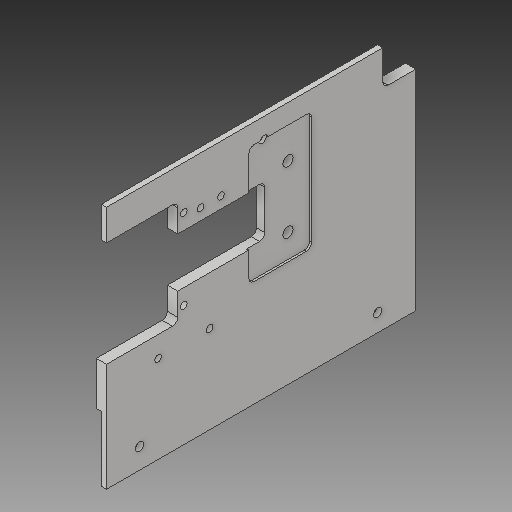
# Autodesk Inventor part: DriveSideBallScrewSupport
Saved by Autodesk Inventor 2018 (Build 220112000, 112)
## iProperties
Created: 2017-10-24
Part Number: DriveSideBallScrewSupport
Material: Generic
Document SubType Name: Modeling
Designer: m228540
Density: 1 g/cm^3
Appearance: Default
Author: m228540
Autodesk Inventor part; units mm, degrees
ref_plane "YZ Plane" through (0, 0, 0) normal (1, 0, 0) x (0, 1, 0)
ref_plane "XZ Plane" through (0, 0, 0) normal (0, 1, 0) x (-1, 0, 0)
ref_plane "XY Plane" through (0, 0, 0) normal (0, 0, 1) x (1, 0, 0)
sketch "Sketch1" plane through (0, 0, 0) normal (1, 0, 0) x (0, 1, 0)
  line L0 (118.5, 150) -> (-118.5, 150)
  line L1 (-118.5, 150) -> (-118.5, -150)
  line L2 (-118.5, -150) -> (118.5, -150)
  line L3 (118.5, -150) -> (118.5, 150)
  line L4 (118.5, 150) -> (-118.5, -150) construction
  line L5 (-118.5, 150) -> (118.5, -150) construction
  point P0 (0, 0)
  dimension "d0" = 300
  dimension "d1" = 237
  constraints: 12 end point, 2 midpoint, 2 parallel, 1 horizontal, 1 perpendicular
  measures "d0" distance of L0.end L1.end
  measures "d1" distance of L1.end L2.end
extrude "Extrusion1" add sketch "Sketch1" along normal mid plane 10
sketch "Sketch2" plane through (5, 0, 0) normal (1, 0, 0) x (0, 0, -1)
  line L0 (150, -118.5) -> (150, 118.5) projected
  line L1 (150, 118.5) -> (118, 118.5)
  line L2 (118, 118.5) -> (118, 89.5)
  line L3 (123, 84.5) -> (150, 84.5)
  line L4 (150, 84.5) -> (150, 118.5)
  arc A0 (118, 89.5) -> (123, 84.5) centre (123, 89.5) ccw
  point P0 (0, 0)
  point P1 (118, 84.5)
  dimension "d4" = 32
  dimension "d5" = 34
  dimension "d6" = 5
  constraints: 8 end point, 2 parallel, 2 point on circle, 2 point on line, 2 tangent, 1 centre point, 1 horizontal, 1 perpendicular
  measures "d4" distance of point (118, 84.5) L3.end
  measures "d5" distance of L1.end point (118, 84.5)
  measures "d6" radius of A0
extrude "Extrusion2" cut sketch "Sketch2" against normal through all
sketch "Sketch3" plane through (5, 0, 0) normal (1, 0, 0) x (0, 0, -1)
  line L0 (-7, -15.5) -> (44, -15.5)
  line L1 (49, -10.5) -> (49, 94.5)
  line L2 (44, 99.5) -> (-7, 99.5)
  line L3 (-12, 94.5) -> (-12, -10.5)
  line L4 (-12, -15.5) -> (49, 99.5) construction
  line L5 (49, -15.5) -> (-12, 99.5) construction
  line L6 (-150, 118.5) -> (-150, -118.5) projected
  line L7 (118, 118.5) -> (-150, 118.5) projected
  arc A0 (-7, 99.5) -> (-12, 94.5) centre (-7, 94.5) ccw
  arc A1 (49, 94.5) -> (44, 99.5) centre (44, 94.5) ccw
  arc A2 (44, -15.5) -> (49, -10.5) centre (44, -10.5) ccw
  arc A3 (-12, -10.5) -> (-7, -15.5) centre (-7, -10.5) ccw
  point P0 (0, 0)
  point P1 (18.5, 42)
  dimension "d9" = 138
  dimension "d10" = 115
  dimension "d11" = 61
  dimension "d12" = 19
  dimension "d13" = 5
  constraints: 12 end point, 8 point on circle, 8 point on line, 8 tangent, 4 centre point, 3 equal radius, 2 midpoint, 2 parallel, 1 horizontal, 1 perpendicular
  measures "d9" distance between parallel lines of L6 L3
  measures "d10" distance of L5.end L4.start
  measures "d11" distance of L4.end L5.end
  measures "d12" distance between parallel lines of L7 L2
  measures "d13" radius of A0
extrude "Extrusion3" cut sketch "Sketch3" against normal blind 2
sketch "Sketch4" plane through (5, 0, 0) normal (1, 0, 0) x (0, 0, -1)
  circle A0 centre (-118, -98.5) radius 4
  circle A1 centre (113, -101.5) radius 4
  circle A2 centre (3, 98.5) radius 4
  line L0 (-150, -118.5) -> (-150, 118.5) projected
  line L1 (-150, -118.5) -> (150, -118.5) projected
  line L2 (150, -118.5) -> (150, 84.5) projected
  line L3 (118, 118.5) -> (-150, 118.5) projected
  point P0 (0, 0)
  dimension "d16" = 8
  dimension "d17" = 32
  dimension "d18" = 20
  dimension "d19" = 17
  dimension "d20" = 37
  dimension "d21" = 153
  dimension "d22" = 20
  constraints: 3 centre point, 2 equal radius
  measures "d16" diameter of A0
  measures "d17" distance from line of L0 A0.centre
  measures "d18" distance from line of L1 A0.centre
  measures "d19" distance from line of L1 A1.centre
  measures "d20" distance from line of L2 A1.centre
  measures "d21" distance from line of L0 A2.centre
  measures "d22" distance from line of L3 A2.centre
extrude "Extrusion4" cut sketch "Sketch4" against normal through all
sketch "Sketch5" plane through (-5, 0, 0) normal (-1, 0, 0) x (0, 0, 1)
  line L0 (150, -118.5) -> (-150, -118.5) projected
  line L1 (-150, -118.5) -> (-83, -118.5)
  line L2 (-83, -118.5) -> (-83, -55.5)
  line L3 (-83, -55.5) -> (-150, -55.5)
  line L4 (-150, -55.5) -> (-150, -118.5)
  line L5 (150, -118.5) -> (80, -118.5)
  line L6 (80, -118.5) -> (80, -55.5)
  line L7 (80, -55.5) -> (150, -55.5)
  line L8 (150, -55.5) -> (150, -118.5)
  line L9 (-118, 118.5) -> (150, 118.5) projected
  line L10 (-150, 84.5) -> (-123, 84.5) projected
  line L11 (150, 118.5) -> (-123, 118.5)
  line L12 (-123, 118.5) -> (-123, 84.5)
  line L13 (-123, 84.5) -> (150, 84.5)
  line L14 (150, 84.5) -> (150, 118.5)
  point P0 (0, 0)
  dimension "d25" = 70
  dimension "d26" = 63
  dimension "d27" = 63
  dimension "d28" = 67
  constraints: 24 end point, 6 parallel, 3 horizontal, 3 perpendicular
  measures "d25" distance of L6.end L7.end
  measures "d26" distance of L5.end L6.end
  measures "d27" distance of L1.end L2.end
  measures "d28" distance of L2.end L3.end
extrude "Extrusion5" cut sketch "Sketch5" against normal blind 5
sketch "Sketch6" plane through (3, 0, 0) normal (1, 0, 0) x (0, 0, -1)
  circle A0 centre (28, 67.5) radius 5
  circle A1 centre (28, 7.5) radius 5
  line L0 (150, -118.5) -> (150, 84.5) projected
  line L1 (118, 118.5) -> (-150, 118.5) projected
  point P0 (0, 0)
  dimension "d31" = 122
  dimension "d32" = 10
  dimension "d34" = 60
  dimension "d35" = 51
  constraints: 2 centre point, 1 equal radius, 1 vertical alignment
  measures "d31" distance from line of L0 A0.centre
  measures "d32" diameter of A0
  measures "d34" distance of A1.centre A0.centre
  measures "d35" distance from line of L1 A0.centre
extrude "Extrusion6" cut sketch "Sketch6" against normal through all
fillet "Fillet1" radius 5 2 edges at (-2.5, -55.5, 80) (-2.5, -55.5, -83)
sketch "Sketch7" plane through (5, 0, 0) normal (1, 0, 0) x (0, 0, -1)
  line L0 (-150, 118.5) -> (-150, -118.5) projected
  line L1 (-150, 88.5) -> (-81, 88.5)
  line L2 (-81, -13.5) -> (-150, -13.5)
  line L3 (-150, -13.5) -> (-150, 88.5)
  line L4 (118, 118.5) -> (-150, 118.5) projected
  line L5 (-81, 102.5) -> (-81, 62.1221) projected
  line L6 (-69, 62.1221) -> (-69, 102.5) projected
  line L7 (15.5, -2.5) -> (15.5, 77.5) projected
  line L8 (-81, 61.5) -> (5.5, 61.5)
  line L9 (5.5, 61.5) -> (5.5, 13.5)
  line L10 (5.5, 13.5) -> (-81, 13.5)
  line L11 (-81, 88.5) -> (-81, 61.5)
  line L12 (-81, 13.5) -> (-81, -13.5)
  point P0 (0, 0)
  dimension "d39" = 30
  dimension "d40" = 102
  dimension "d41" = 57
  dimension "d42" = 10
  dimension "d43" = 48
  constraints: 16 end point, 4 parallel, 3 perpendicular, 2 collinear, 2 horizontal, 2 point on line
  measures "d39" distance between parallel lines of L4 L1
  measures "d40" distance of L1.end L2.start
  measures "d41" distance between parallel lines of L8 L4
  measures "d42" distance between parallel lines of L9 L7
  measures "d43" distance of L8.end L9.end
extrude "Extrusion7" cut sketch "Sketch7" against normal through all
fillet "Fillet2" radius 5 4 edges at (2.5, 88.5, 81) (0, -13.5, 81) (-1, 13.5, -5.5) (-1, 61.5, -5.5)
sketch "Sketch8" plane through (5, 0, 0) normal (1, 0, 0) x (0, 0, -1)
  circle A0 centre (-100, -33.5) radius 3 construction
  circle A1 centre (-50, -33.5) radius 3 construction
  circle A2 centre (-59, 72.5) radius 3 construction
  circle A3 centre (-39, 72.5) radius 3 construction
  circle A4 centre (-75, 76.5) radius 3 construction
  circle A5 centre (-75, -1.5) radius 3 construction
  circle A6 centre (-75, 76.5) radius 3.25
  circle A7 centre (-59, 72.5) radius 3.25
  circle A8 centre (-39, 72.5) radius 3.25
  circle A9 centre (-75, -1.5) radius 3.25
  circle A10 centre (-50, -33.5) radius 3.25
  circle A11 centre (-100, -33.5) radius 3.25
  point P0 (0, 0)
  dimension "d49" = 0.25
  dimension "d50" = 0.25
  dimension "d51" = 0.25
  dimension "d52" = 0.25
  dimension "d53" = 0.25
  dimension "d54" = 0.25
  constraints: 6 centre point
  measures "d49" radial gap between concentric circles of A4 A6
  measures "d50" radial gap between concentric circles of A2 A7
  measures "d51" radial gap between concentric circles of A3 A8
  measures "d52" radial gap between concentric circles of A5 A9
  measures "d53" radial gap between concentric circles of A1 A10
  measures "d54" radial gap between concentric circles of A0 A11
extrude "Extrusion8" cut sketch "Sketch8" against normal through all
body "Solid1"
